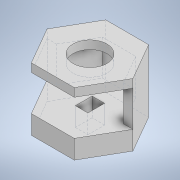
# Autodesk Inventor part: encoder_magnet_socket
Saved by Autodesk Inventor 2021 (Build 250183000, 183)
## iProperties
Created: 2020-12-10
Part Number: encoder_magnet_socket
Material: Generic
Document SubType Name: Modeling
Designer: Mateusz
Density: 1 g/cm^3
Appearance: Default
Author: Mateusz
Autodesk Inventor part; units mm, degrees
ref_plane "YZ Plane" through (0, 0, 0) normal (1, 0, 0) x (0, 1, 0)
ref_plane "XZ Plane" through (0, 0, 0) normal (0, 1, 0) x (-1, 0, 0)
ref_plane "XY Plane" through (0, 0, 0) normal (0, 0, 1) x (1, 0, 0)
sketch "Sketch1" plane through (0, 0, 0) normal (0, 1, 0) x (-1, 0, 0)
  circle A0 centre (0, 0) radius 4.05
  line L0 (0, 0) -> (7.25, 0)
  line L1 (7.25, 0) -> (3.625, -6.2787)
  line L2 (3.625, -6.2787) -> (-3.625, -6.2787)
  line L3 (-3.625, -6.2787) -> (-7.25, 0)
  line L4 (-7.25, 0) -> (-3.625, 6.2787)
  line L5 (-3.625, 6.2787) -> (3.625, 6.2787)
  line L6 (3.625, 6.2787) -> (7.25, 0)
  line L7 (7.25, 0) -> (10.25, 0)
  line L8 (10.25, 0) -> (5.125, -8.8768)
  line L9 (5.125, -8.8768) -> (-5.125, -8.8768)
  line L10 (-5.125, -8.8768) -> (-10.25, 0)
  line L11 (-10.25, 0) -> (-5.125, 8.8768)
  line L12 (-5.125, 8.8768) -> (5.125, 8.8768)
  line L13 (5.125, 8.8768) -> (10.25, 0)
  line L14 (-7.25, 0) -> (-10.25, 0)
  point P0 (0, 0)
  point P1 (-10.25, 0)
  dimension "d0" = 8.1
  dimension "d1" = 7.25
  dimension "d2" = 3
  constraints: 30 end point, 2 coincident, 2 horizontal, 1 centre point, 1 point on line, 26 other
  measures "d0" diameter of A0
  measures "d1" distance of L0.start L0.end
  measures "d2" distance of L0.end L7.end
extrude "Extrusion1" add sketch "Sketch1" along normal blind 2
extrude "Extrusion2" add sketch "Sketch1" against normal blind 8 contours L7 L8 L9 L10 L14 L3 L2 L1
sketch "Sketch2" plane through (0, -8, 0) normal (0, -1, 0) x (1, 0, 0)
  circle A0 centre (0, 0) radius 4.05 projected
  line L0 (-10.25, 0) -> (-7.25, 0) projected
  line L1 (-7.25, 0) -> (-3.625, -6.2787) projected
  line L2 (-3.625, -6.2787) -> (3.625, -6.2787) projected
  line L3 (3.625, -6.2787) -> (7.25, 0) projected
  line L4 (7.25, 0) -> (10.25, 0) projected
  line L5 (5.125, 8.8768) -> (10.25, 0) projected
  line L6 (-5.125, 8.8768) -> (5.125, 8.8768) projected
  line L7 (-10.25, 0) -> (-5.125, 8.8768) projected
  line L8 (3.625, -6.2787) -> (-3.625, -6.2787) projected
  line L9 (-3.625, -6.2787) -> (-7.25, 0) projected
  line L10 (-7.25, 0) -> (-10.25, 0) projected
  line L11 (-10.25, 0) -> (-5.125, -8.8768) projected
  line L12 (-5.125, -8.8768) -> (5.125, -8.8768) projected
  line L13 (5.125, -8.8768) -> (10.25, 0) projected
  line L14 (10.25, 0) -> (7.25, 0) projected
  line L15 (7.25, 0) -> (3.625, -6.2787) projected
  line L16 (3.625, 6.2787) -> (-3.625, 6.2787) projected
  line L17 (-3.625, 6.2787) -> (-7.25, 0) projected
  line L18 (7.25, 0) -> (3.625, 6.2787) projected
extrude "Extrusion3" add sketch "Sketch2" along normal blind 5 contours A0 | L7 L6 L5 L4 L18 L16 L17 L0 | L0 L1 L2 L3 L4 L13 L12 L11 | L17 L16 L18 L3 L2 L1
sketch "Sketch3" plane through (0, -13, 0) normal (0, -1, 0) x (1, 0, 0)
  line L0 (0, 0) -> (1.5, 0)
  line L1 (1.5, 0) -> (-1.5, 0)
  line L2 (1.5, 0) -> (1.5, 2)
  line L3 (1.5, 2) -> (-1.5, 2)
  line L4 (-1.5, 2) -> (-1.5, -2)
  line L5 (-1.5, -2) -> (1.5, -2)
  line L6 (1.5, -2) -> (1.5, 0)
  line L7 (5.125, 8.8768) -> (-5.125, 8.8768) projected
  line L8 (-5.125, 8.8768) -> (-10.25, 0) projected
  line L9 (-10.25, 0) -> (-5.125, -8.8768) projected
  line L10 (-5.125, -8.8768) -> (5.125, -8.8768) projected
  line L11 (5.125, -8.8768) -> (10.25, 0) projected
  line L12 (10.25, 0) -> (5.125, 8.8768) projected
  dimension "d9" = 1.5
  dimension "d10" = 3
  dimension "d11" = 2
  dimension "d12" = 3
  dimension "d13" = 4
  constraints: 14 end point, 5 perpendicular, 2 point on line, 1 horizontal
  measures "d9" distance of L0.start L0.end
  measures "d10" distance of L0.end L1.end
  measures "d11" distance of L0.end L2.end
  measures "d12" distance of L2.end L3.end
  measures "d13" distance of L3.end L4.end
extrude "Extrusion4" cut sketch "Sketch3" against normal blind 4.5 contours L1 L4 L3 L2 L0 | L0 L6 L5 L4 L1
sketch "Sketch5" plane through (0, -8, 0) normal (0, 1, 0) x (1, 0, 0)
  circle A0 centre (0, 0) radius 4.05 projected
  line L0 (-10.25, 0) -> (-7.25, 0) projected
  line L1 (-7.25, 0) -> (-3.625, 6.2787) projected
  line L2 (-3.625, 6.2787) -> (3.625, 6.2787) projected
  line L3 (3.625, 6.2787) -> (7.25, 0) projected
  line L4 (7.25, 0) -> (10.25, 0) projected
  line L5 (5.125, -8.8768) -> (10.25, 0) projected
  line L6 (-5.125, -8.8768) -> (5.125, -8.8768) projected
  line L7 (-10.25, 0) -> (-5.125, -8.8768) projected
  line L8 (3.625, 6.2787) -> (-3.625, 6.2787) projected
  line L9 (3.625, 6.2787) -> (4, 6.9282)
  line L10 (4, 6.9282) -> (8, 0)
  line L11 (8, 0) -> (4, -6.9282)
  line L12 (4, -6.9282) -> (-4, -6.9282)
  line L13 (-4, -6.9282) -> (-8, 0)
  line L14 (-8, 0) -> (-4, 6.9282)
  line L15 (-4, 6.9282) -> (4, 6.9282)
  point P0 (8, 0)
  point P1 (-8, 0)
  dimension "d19" = 0.75
  constraints: 14 end point, 1 coincident, 13 other
  measures "d19" distance of L2.end L9.end
extrude "Extrusion6" cut sketch "Sketch5" along normal up to surface (8 mm away) contours L14 L15 L9 L2 L1 L0 | L10 L4 L3 L9
sketch "Sketch6" plane through (0, -8, 0) normal (0, 1, 0) x (1, 0, 0)
  line L0 (-8, 0) -> (-10.25, 0) projected
  line L1 (-5.125, -8.8768) -> (-10.25, 0) projected
  line L2 (5.125, -8.8768) -> (-5.125, -8.8768) projected
  line L3 (10.25, 0) -> (5.125, -8.8768) projected
  line L4 (10.25, 0) -> (8, 0) projected
  line L5 (8, 0) -> (4, 6.9282) projected
  line L6 (4, 6.9282) -> (-4, 6.9282) projected
  line L7 (-4, 6.9282) -> (-8, 0) projected
  point P0 (0, 0)
extrude "Extrusion7" cut sketch "Sketch6" against normal up to surface (0.5 mm away)
body "Solid1"
